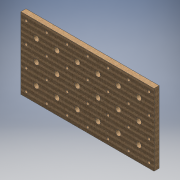
# Autodesk Inventor part: BearingSiliconeMold_1
Saved by Autodesk Inventor 2016 (Build 200138000, 138)
## iProperties
Created: 2015-12-06
Part Number: BearingSiliconeMold_1
Material: MDF Medium Density Fiberboard
Document SubType Name: Modeling
Designer: DonMo
Density: 0.8 g/cm^3
Appearance: Cardboard - Corrugated
Author: DonMo
Autodesk Inventor part; units mm, degrees
ref_plane "YZ Plane" through (0, 0, 0) normal (1, 0, 0) x (0, 1, 0)
ref_plane "XZ Plane" through (0, 0, 0) normal (0, 1, 0) x (-1, 0, 0)
ref_plane "XY Plane" through (0, 0, 0) normal (0, 0, 1) x (1, 0, 0)
sketch "Sketch1" plane through (0, 0, 0) normal (0, 1, 0) x (-1, 0, 0)
  circle A0 centre (0, 0) radius 9 construction
  circle A1 centre (0, 0) radius 7 construction
  circle A2 centre (12, -12) radius 1.715
  line L0 (0, 0) -> (0, -7) construction
  line L1 (0, 0) -> (9, 0) construction
  circle A3 centre (0, 0) radius 3.175
  line L2 (18, -66) -> (-138, -66)
  line L3 (-138, -66) -> (-138, 18)
  line L4 (-138, 18) -> (18, 18)
  line L5 (18, 18) -> (18, -66)
  circle A4 centre (12, 12) radius 1.715
  circle A5 centre (-12, 12) radius 1.715
  circle A6 centre (-12, -12) radius 1.715
  line L6 (12, -12) -> (0, 0) construction
  circle A7 centre (0, -24) radius 3.175
  circle A8 centre (12, -36) radius 1.715
  circle A9 centre (-12, -36) radius 1.715
  circle A10 centre (0, -48) radius 3.175
  circle A11 centre (12, -60) radius 1.715
  circle A12 centre (-12, -60) radius 1.715
  circle A13 centre (-36, 12) radius 1.715
  circle A14 centre (-24, 0) radius 3.175
  circle A15 centre (-36, -12) radius 1.715
  circle A16 centre (-24, -24) radius 3.175
  circle A17 centre (-36, -36) radius 1.715
  circle A18 centre (-24, -48) radius 3.175
  circle A19 centre (-36, -60) radius 1.715
  circle A20 centre (-60, 12) radius 1.715
  circle A21 centre (-48, 0) radius 3.175
  circle A22 centre (-60, -12) radius 1.715
  circle A23 centre (-48, -24) radius 3.175
  circle A24 centre (-60, -36) radius 1.715
  circle A25 centre (-48, -48) radius 3.175
  circle A26 centre (-60, -60) radius 1.715
  circle A27 centre (-84, 12) radius 1.715
  circle A28 centre (-72, 0) radius 3.175
  circle A29 centre (-84, -12) radius 1.715
  circle A30 centre (-72, -24) radius 3.175
  circle A31 centre (-84, -36) radius 1.715
  circle A32 centre (-72, -48) radius 3.175
  circle A33 centre (-84, -60) radius 1.715
  circle A34 centre (-108, 12) radius 1.715
  circle A35 centre (-96, 0) radius 3.175
  circle A36 centre (-108, -12) radius 1.715
  circle A37 centre (-96, -24) radius 3.175
  circle A38 centre (-108, -36) radius 1.715
  circle A39 centre (-96, -48) radius 3.175
  circle A40 centre (-108, -60) radius 1.715
  circle A41 centre (-132, 12) radius 1.715
  circle A42 centre (-120, 0) radius 3.175
  circle A43 centre (-132, -12) radius 1.715
  circle A44 centre (-120, -24) radius 3.175
  circle A45 centre (-132, -36) radius 1.715
  circle A46 centre (-120, -48) radius 3.175
  circle A47 centre (-132, -60) radius 1.715
  dimension "d0" = 18
  dimension "d1" = 2
  dimension "d2" = 3.43
  dimension "d6" = 6.35
  dimension "d27" = 360
  dimension "d29" = 45
  dimension "d30" = 12
  dimension "d33" = 24
  dimension "d40" = 24
  dimension "d45" = 6
  dimension "d46" = 6
  dimension "d47" = 6
  dimension "d48" = 6
  constraints: 46 centre point, 14 end point, 3 coincident, 3 horizontal, 2 parallel, 2 vertical, 1 horizontal alignment, 1 perpendicular, 1 vertical alignment, 95 other
  measures "d2" diameter of A2
  measures "d6" diameter of A3
  measures "d29" angle of L0 L6
  measures "d30" horizontal distance of L6.start point (0, 0)
  measures "d33" distance of L6.end A7.centre
  measures "d40" distance of A5.centre A13.centre
  measures "d45" distance from line of A4.centre L4
  measures "d46" distance from line of L5 A4.centre
  measures "d47" distance from line of L2 A11.centre
  measures "d48" distance from line of A41.centre L3
extrude "Extrusion3" add sketch "Sketch1" along normal blind 5.95
equation "\"d0\" = 0.75 * BearingDiameter"
equation "\"d1\" = SiliconeOverlapThickness"
equation "\"d2\" = HoldScrewDiameter"
equation "\"d6\" = DowlDiameter"
equation "\"d49\" = WoodThickness"
equation "\"BearingDiameter\" = 24"
equation "\"SiliconeOverlapThickness\" = 2"
equation "\"HoldScrewDiameter\" = 3.43"
equation "\"DowlDiameter\" = 6.35"
equation "\"WoodThickness\" = 5.95"
body "Solid3"
